LED Light Holder Middle (Autodesk Fusion 360 design; units mm, degrees)
Autodesk Fusion 360 part; units mm, degrees
box "BoxPrimitive1" add length 200 width 30 height 5 placed x (0, 0, -1) y (-1, 0, 0) z (0, 1, 0) at (20, 0, 130) in component "Component"
sketch "Sketch2" plane through (0, 5, 0) normal (0, 1, 0) x (-1, 0, 0) in component "Component"
  line L0 (-20, -70) -> (10, -70)
  line L1 (10, -70) -> (10, 130)
  line L2 (10, 130) -> (-20, 130)
  line L3 (-20, 130) -> (-20, -70)
  point P0 (-15, -65)
  point P1 (5, -65)
  point P2 (-15, 125)
  point P3 (5, 125)
  dimension "d19" = 20
  dimension "d20" = 5
  dimension "d21" = 5
  dimension "d22" = 5
  constraint horizontal P2 P3
  constraint horizontal P0 P1
  constraint vertical P1 P3
  constraint vertical P0 P2
  measures "d19" distance of P2 P3
  measures "d20" distance of L3 P2
  measures "d21" distance of L2 P2
  measures "d22" distance of L0 P0
hole "Hole1" at (15, 5, -65) at (-5, 5, -65) at (-5, 5, 125) at (15, 5, 125) direction (0, -1, 0) diameter 3.4 depth 12 tip angle 118 countersink diameter 6.3 countersink angle 90 in component "Component"
extrude "Extrude1" cut 1 faces at (8.2675, 0, -1.0962) along direction (0, 1, 0) blind 2.5 in component "Component"
extrude "Extrude2" cut 1 faces at (8.2675, 2.5, -1.0962) along direction (0, 1, 0) blind 0.1 in component "Component"
component "Component" placed x (1, 0, 0) y (0, 1, 0) z (0, 0, 1) at (0, 0, 0)
